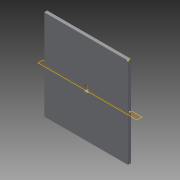
# Autodesk Inventor part: socle
Saved by Autodesk Inventor 2015 (Build 190159000, 159)
## iProperties
Created: 2015-02-16
Part Number: socle
Material: Générique
Document SubType Name: Modeling
Designer: informatique
Density: 1 g/cm^3
Appearance: Par défaut
Author: informatique
Autodesk Inventor part; units mm, degrees
ref_plane "YZ Plane" through (0, 0, 0) normal (1, 0, 0) x (0, 1, 0)
ref_plane "XZ Plane" through (0, 0, 0) normal (0, 1, 0) x (-1, 0, 0)
ref_plane "XY Plane" through (0, 0, 0) normal (0, 0, 1) x (1, 0, 0)
sketch "Esquisse1" plane through (0, 0, 0) normal (0, 1, 0) x (-1, 0, 0)
  line L0 (0, 0) -> (25.9, 0)
  line L1 (25.9, 0) -> (25.9, -27.9)
  line L2 (25.9, -27.9) -> (0, -27.9)
  line L3 (0, -27.9) -> (0, 0)
  dimension "d0" = 27.9
  dimension "d1" = 25.9
  constraints: 8 end point, 2 parallel, 1 horizontal, 1 perpendicular
  measures "d0" distance of L0.end L1.end
  measures "d1" distance of L1.end L2.end
extrude "Extrusion1" add sketch "Esquisse1" along normal blind 0.45 and the other way blind 0.475
sketch "Esquisse5" plane through (0, -0.475, 0) normal (0, -1, 0) x (1, 0, 0)
  line L0 (-12.65, -12) -> (-13.25, -12)
  line L1 (-13.25, -12) -> (-13.25, -13.9)
  line L2 (-13.25, -13.9) -> (-12.65, -13.9)
  line L3 (-12.65, -13.9) -> (-12.65, -12)
  line L4 (-13.9, -12.65) -> (-12, -12.65)
  line L5 (-12, -12.65) -> (-12, -13.3)
  line L6 (-12, -13.3) -> (-13.9, -13.3)
  line L7 (-13.9, -13.3) -> (-13.9, -12.65)
  line L8 (0, 0) -> (-25.9, 0) projected
  line L9 (0, -27.9) -> (0, 0) projected
  dimension "d18" = 0.65
  dimension "d19" = 0.6
  dimension "d20" = 1.9
  dimension "d21" = 1.9
  dimension "d22" = 0.65
  dimension "d23" = 0.65
  dimension "d24" = 12.65
  dimension "d25" = 12.65
  constraints: 16 end point, 4 parallel, 2 horizontal, 2 perpendicular
  measures "d18" distance of L4.end L5.end
  measures "d19" distance of L1.end L2.end
  measures "d20" distance of L4.start L4.end
  measures "d21" distance of L0.end L1.end
  measures "d22" distance between parallel lines of L5 L3
  measures "d23" distance between parallel lines of L0 L4
  measures "d24" distance between parallel lines of L8 L4
  measures "d25" distance between parallel lines of L9 L3
extrude "Extrusion3" cut sketch "Esquisse5" against normal blind 1000
